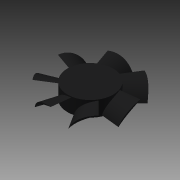
# Autodesk Inventor part: fan_3007_blaze
Saved by Autodesk Inventor 2013 (Build 170138000, 138)
## iProperties
Created: 2014-03-19
Part Number: fan_3007_blaze
Document SubType Name: Modeling
Designer: Noa Izumi
Material: Default
Density: 1 g/cm^3
Control State: 0
Master: False
Checked Out: False
Shininess: 41.0
Density: 0.0
Volumn: 0.0
Area: 0.0
PropertySet Name: Model Information
Author: Noa Izumi
Autodesk Inventor part; units mm, degrees
ref_plane "YZ Plane" through (0, 0, 0) normal (1, 0, 0) x (0, 1, 0)
ref_plane "XZ Plane" through (0, 0, 0) normal (0, 1, 0) x (-1, 0, 0)
ref_plane "Work Plane1" through (14, 0, 0) normal (1, 0, 0) x (0, 0, -1)
sketch "Sketch2" plane through (0, 0, 0) normal (1, 0, 0) x (0, 1, 0)
  arc A0 (1.9695, 4.7202) -> (-2.3191, 0.3527) centre (2.9183, -0.5007) ccw
  arc A1 (1.9695, 4.7202) -> (-2.3191, 0.3527) centre (6.9579, -4.4673) ccw
  constraints: 4 point on circle, 2 centre point
sketch "Sketch5" plane through (14, 0, 0) normal (1, 0, 0) x (0, 0, -1)
  arc A0 (-4.7202, 3.5423) -> (-0.3527, -3.8232) centre (2.3417, 2.7522) ccw
  arc A1 (-4.7202, 3.5423) -> (-0.3527, -3.8232) centre (5.6636, 4.722) ccw
  constraints: 4 point on circle, 2 centre point
loft "Loft1" add profiles "Sketch2", "Sketch5"
sketch "Sketch7" plane through (0, 0, 0) normal (0, 0, 1) x (1, 0, 0)
  circle A0 centre (0, 0) radius 7.5
  dimension "d10" = 15
  constraints: 1 centre point
  measures "d10" diameter of A0
extrude "Extrusion3" add sketch "Sketch7" along normal blind 5
pattern_circular "Circular Pattern1" count 7 over 360 about axis through (0, 0, 0) along (0, 0, 1) of "Loft1"
sketch "Sketch8" plane through (0, 0, 5) normal (0, 0, 1) x (1, 0, 0)
  circle A0 centre (0, 0) radius 7.5 projected
  circle A1 centre (0, 0) radius 13.5
  circle A2 centre (0, 0) radius 15
  dimension "d16" = 27
  dimension "d17" = 30
  constraints: 2 centre point, 2 coincident
  measures "d16" diameter of A1
  measures "d17" diameter of A2
extrude "Extrusion4" cut sketch "Sketch8" against normal blind 5 contours A2
